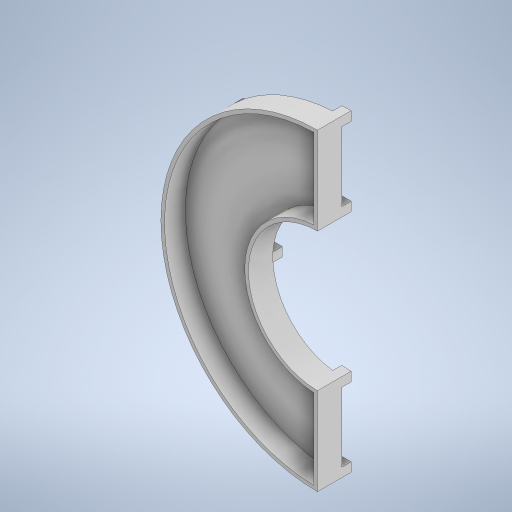
# Autodesk Inventor part: Bandeja Radial
Saved by Autodesk Inventor 2023 (Build 270158000, 158)
## iProperties
Created: 2023-03-08
Part Number: Bandeja Radial
Material: Genérico
Document SubType Name: Modeling
Designer: Inteli
Density: 1 g/cm^3
Appearance: Padrão
Author: Inteli
Autodesk Inventor part; units mm, degrees
ref_plane "YZ Plane" through (0, 0, 0) normal (1, 0, 0) x (0, 1, 0)
ref_plane "XZ Plane" through (0, 0, 0) normal (0, 1, 0) x (-1, 0, 0)
ref_plane "XY Plane" through (0, 0, 0) normal (0, 0, 1) x (1, 0, 0)
sketch "Esboço1" plane through (0, 0, 0) normal (0, 0, 1) x (1, 0, 0)
  arc A0 (0, 340) -> (0, -340) centre (0, 0) ccw
  arc A1 (0, 150) -> (0, -150) centre (0, 0) ccw
  line L0 (0, 0) -> (170, 0) construction
  line L1 (0, 0) -> (155, 0) construction
  line L2 (0, 0) -> (155, 0) construction
  line L3 (0, 340) -> (0, 150)
  line L4 (0, -150) -> (0, -340)
  arc A2 (-8, 157.7973) -> (-8, -157.7973) centre (0, 0) ccw
  line L5 (-8, -157.7973) -> (-8, -331.9036)
  arc A3 (-8, 331.9036) -> (-8, -331.9036) centre (0, 0) ccw
  line L6 (-8, 331.9036) -> (-8, 157.7973)
  dimension "d16" = 680
  dimension "d17" = 300
  dimension "d37" = 8
  constraints: 14 end point, 8 point on circle, 4 centre point, 3 horizontal, 2 coincident, 2 vertical, 3 other
  measures "d16" diameter of A0
  measures "d17" diameter of A1
  measures "d37" distance between parallel lines of L3 L6
extrude "Parede" add sketch "Esboço1" along normal blind 45
extrude "Fundo" add sketch "Esboço1" against normal blind 8 contours L3 A1 L4 A0 | A2 L5 A3 L6
sketch "Esboço3" plane through (0, 0, -8) normal (0, 0, -1) x (-1, 0, 0)
  line L0 (0, 150) -> (0, 170)
  line L1 (0, 340) -> (0, 150) projected
  line L2 (0, 170) -> (20, 170)
  line L3 (20, 170) -> (20, 148.6607)
  arc A0 (20, 148.6607) -> (0, 150) centre (0, 0) ccw
  line L4 (0, 340) -> (0, 320)
  line L5 (0, 320) -> (20, 320)
  arc A1 (0, -340) -> (0, 340) centre (0, 0) ccw projected
  line L6 (20, 320) -> (20, 339.4113)
  arc A2 (20, 339.4113) -> (0, 340) centre (0, 0) ccw
  line L7 (247.3834, 233.2412) -> (233.3452, 219.2031)
  line L8 (233.2412, 247.3834) -> (219.2031, 233.3452)
  arc A3 (233.3452, 219.2031) -> (219.2031, 233.3452) centre (0.1105, 0.1105) ccw
  arc A4 (247.3834, 233.2412) -> (233.2412, 247.3834) centre (0, 0) ccw
  line L9 (0, -150) -> (0, -170)
  line L10 (0, -340) -> (0, -150)
  line L11 (0, -170) -> (20, -170)
  line L12 (20, -170) -> (20, -148.6607)
  arc A5 (0, -150) -> (20, -148.6607) centre (0, 0) ccw
  line L13 (0, -340) -> (0, -320)
  line L14 (0, -320) -> (20, -320)
  line L15 (20, -320) -> (20, -339.4113)
  arc A6 (0, -340) -> (20, -339.4113) centre (0, 0) ccw
  line L16 (170, 0) -> (170, -10)
  line L17 (170, -10) -> (149.6663, -10)
  line L18 (170, 0) -> (170, 10)
  line L19 (170, 10) -> (149.6648, 10.0224)
  arc A7 (149.6663, -10) -> (149.6648, 10.0224) centre (0, 0) ccw
  line L20 (320, 0) -> (320, -10)
  line L21 (320, 0) -> (320, 10)
  line L22 (320, 10) -> (339.8529, 10)
  line L23 (320, -10) -> (339.8529, -10)
  arc A8 (339.8529, -10) -> (339.8529, 10) centre (0, 0) ccw
  line L24 (247.3834, -233.2412) -> (233.3452, -219.2031)
  line L25 (233.2412, -247.3834) -> (219.2031, -233.3452)
  arc A9 (219.2031, -233.3452) -> (233.3452, -219.2031) centre (0.1105, -0.1105) ccw
  arc A10 (233.2412, -247.3834) -> (247.3834, -233.2412) centre (0, 0) ccw
  constraints: 50 end point, 25 point on circle, 10 centre point, 5 perpendicular, 4 point on line, 3 vertical, 2 concentric, 1 parallel
extrude "Pé da Bandeja" add sketch "Esboço3" along normal blind 20
